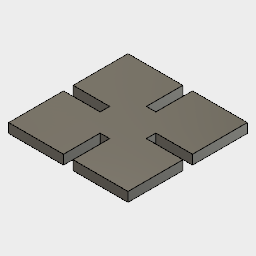
WEEK 3 HOMEWORK v2 (Autodesk Fusion 360 design; units mm, degrees)
Autodesk Fusion 360 part; units mm, degrees
sketch "草图1" plane through (0, 0, 0) normal (0, 1, 0) x (1, 0, 0) in component "module 1"
  line L0 (0, 0) -> (15, 0)
  line L1 (15, 0) -> (15, -10)
  line L2 (15, -10) -> (17.6, -10)
  line L3 (17.6, -10) -> (17.6, 0)
  line L4 (17.6, 0) -> (32.6, 0)
  line L5 (32.6, 0) -> (32.6, -15)
  line L6 (32.6, -15) -> (22.6, -15)
  line L7 (22.6, -15) -> (22.6, -17.6)
  line L8 (22.6, -17.6) -> (32.6, -17.6)
  line L9 (32.6, -17.6) -> (32.6, -32.6)
  line L10 (32.6, -32.6) -> (17.6, -32.6)
  line L11 (17.6, -32.6) -> (17.6, -22.6)
  line L12 (17.6, -22.6) -> (15, -22.6)
  line L13 (15, -22.6) -> (15, -32.6)
  line L14 (15, -32.6) -> (0, -32.6)
  line L15 (0, -32.6) -> (0, -17.6)
  line L16 (0, -17.6) -> (10, -17.6)
  line L17 (10, -17.6) -> (10, -15)
  line L18 (10, -15) -> (0, -15)
  line L19 (0, -15) -> (0, 0)
  dimension "d17" = 15
  dimension "d18" = 10
  dimension "d19" = 2.6
  dimension "d20" = 10
  dimension "d21" = 15
  dimension "d22" = 15
  dimension "d23" = 10
  dimension "d24" = 2.6
  dimension "d25" = 10
  dimension "d26" = 15
  dimension "d27" = 15
  dimension "d28" = 10
  dimension "d29" = 2.6
  dimension "d30" = 10
  dimension "d31" = 15
  dimension "d32" = 15
  dimension "d33" = 10
  dimension "d34" = 2.6
  dimension "d35" = 10
  dimension "d36" = 15
  measures "d17" distance of L0.start L0.end
  measures "d18" distance of L0.end L1.end
  measures "d19" distance of L1.end L2.end
  measures "d20" distance of L2.end L3.end
  measures "d21" distance of L3.end L4.end
  measures "d22" distance of L4.end L5.end
  measures "d23" distance of L5.end L6.end
  measures "d24" distance of L6.end L7.end
  measures "d25" distance of L7.end L8.end
  measures "d26" distance of L8.end L9.end
  measures "d27" distance of L9.end L10.end
  measures "d28" distance of L10.end L11.end
  measures "d29" distance of L11.end L12.end
  measures "d30" distance of L12.end L13.end
  measures "d31" distance of L13.end L14.end
  measures "d32" distance of L14.end L15.end
  measures "d33" distance of L15.end L16.end
  measures "d34" distance of L16.end L17.end
  measures "d35" distance of L17.end L18.end
  measures "d36" distance of L18.end L0.start
extrude "Extrude1" add sketch "草图1" along normal blind 2.6
component "module 1" placed x (1, 0, 0) y (0, 1, 0) z (0, 0, 1) at (0, 0, 0)
equation "edge = 15 mm" comment "outward"
equation "fit = 2.6 mm"
equation "cut = 10 mm"
equation "d17 = edge"
equation "d18 = cut"
equation "d19 = fit"
equation "d20 = cut"
equation "d21 = edge"
equation "d22 = edge"
equation "d23 = cut"
equation "d24 = fit"
equation "d25 = cut"
equation "d26 = edge"
equation "d27 = edge"
equation "d28 = cut"
equation "d29 = fit"
equation "d30 = cut"
equation "d31 = edge"
equation "d32 = edge"
equation "d33 = cut"
equation "d34 = fit"
equation "d35 = cut"
equation "d36 = edge"
equation "d37 = fit"
